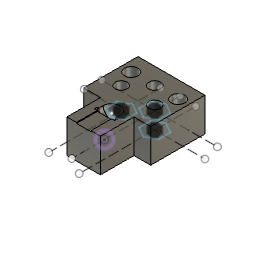
bending_tool_lower_LED v7 (Autodesk Fusion 360 design; units mm, degrees)
Autodesk Fusion 360 part; units mm, degrees
sketch "Skizze1" plane through (0, 0, 0) normal (0, 0, 1) x (1, 0, 0)
  line L0 (-3, 0) -> (-3, 0.8)
  line L1 (-3, 0.8) -> (-2.5, 0.8)
  line L2 (-2.5, 0.8) -> (-2.5, 2.1)
  line L3 (-8.4843, 2.1) -> (11.6981, 2.1) construction
  line L4 (0, 9) -> (0, -6.2163) construction
  arc A0 (0, 4.6) -> (-2.5, 2.1) centre (0, 2.1) ccw
  line L5 (0, 4.6) -> (0, 0)
  line L6 (0, 0) -> (-3, 0)
  line L7 (2.5, 2) -> (4.5, 2)
  line L8 (4.5, 2) -> (4.5, -2)
  line L9 (4.5, -2) -> (2.5, -2)
  line L10 (2.5, -2) -> (2.5, 2)
  line L11 (-4.5, 2) -> (-2.5, 2)
  line L12 (-2.5, 2) -> (-2.5, -2)
  line L13 (-2.5, -2) -> (-4.5, -2)
  line L14 (-4.5, -2) -> (-4.5, 2)
  point P0 (0, 2.1)
  dimension "d1" = 3
  dimension "d2" = 0.8
  dimension "d3" = 2.5
  dimension "d7" = 2.5
  dimension "d8" = 2
  dimension "d9" = 2
  dimension "d10" = 2
  dimension "d117" = 2.5
  dimension "d119" = 2
  dimension "d120" = 2
  dimension "d121" = 2
  dimension "d122" = 2.1
  dimension "d123" = 4.6
  constraint vertical L0
  constraint perpendicular L0 L1
  constraint perpendicular L1 L2
  constraint horizontal L3
  constraint perpendicular L3 L4
  constraint coincident L5.end L4
  constraint coincident L4 P0
  constraint coincident L3 P0
  constraint coincident L4 A0.start
  constraint coincident P0 A0.centre
  constraint coincident L5.end L6.start
  constraint perpendicular L0 L6
  constraint horizontal L7
  constraint vertical L8
  constraint horizontal L9
  constraint vertical L10
  constraint horizontal L11
  constraint vertical L12
  constraint horizontal L13
  constraint vertical L14
  constraint coincident L2.end L3
  measures "d1" distance of L5.end L0
  measures "d2" distance of L0.start L0.end
  measures "d3" distance of L5.end L2
  measures "d7" distance of L5.end L10
  measures "d8" vertical distance of L5.end L7.start
  measures "d9" distance of L5.end L9
  measures "d10" distance of L8 L10
  measures "d117" distance of L5.end L12
  measures "d119" distance of L12 L14
  measures "d120" distance of L5.end L13
  measures "d121" distance of L5.end L11
  measures "d122" distance of L5.end L3
  measures "d123" distance of L5.end A0.start
revolve "Drehen1" add sketch "Skizze1" angle 360 about axis through (0, 9, 0) along (0, -1, 0) contours L0 L1 L6 L12 | L2 A0 L5 L6 L12 makes body 1
sketch "Skizze2" plane through (0, 0, 0) normal (0, 0, 1) x (1, 0, 0)
  line L0 (-10, 20) -> (10, 20)
  line L1 (10, 20) -> (10, -6.2)
  line L2 (10, -6.2) -> (-10, -6.2)
  line L3 (-10, -6.2) -> (-10, 20)
  line L4 (0, 21.3723) -> (0, -17) construction
  line L5 (-26.2349, 0) -> (38.3962, 0) construction
  line L6 (5, -6.2) -> (5, 3.8)
  line L7 (5, 3.8) -> (10, 3.8)
  line L8 (-5, -6.2) -> (-5, 3.8)
  line L9 (-5, 3.8) -> (-10, 3.8)
  line L10 (-17, 10) -> (24.4562, 10) construction
  line L11 (-5, 26) -> (-5, 5) construction
  line L12 (5, 25.6741) -> (5, 5) construction
  circle A0 centre (-5, 10) radius 1.75
  circle A1 centre (5, 10) radius 1.75
  line L13 (-16, 15) -> (36.57, 15) construction
  circle A2 centre (0, 15) radius 1.75
  line L14 (-7, 22.2425) -> (-7, -4.6464) construction
  line L15 (7, 22.2425) -> (7, -3.3633) construction
  circle A3 centre (-7, 15) radius 2
  circle A4 centre (7, 15) radius 2
  dimension "d13" = 10
  dimension "d14" = 10
  dimension "d15" = 6.2
  dimension "d16" = 20
  dimension "d32" = 5
  dimension "d33" = 10
  dimension "d34" = 5
  dimension "d35" = 10
  dimension "d36" = 10
  dimension "d37" = 5
  dimension "d38" = 5
  dimension "d39" = 3.5
  dimension "d40" = 3.5
  dimension "d41" = 5
  dimension "d42" = 3.5
  dimension "d53" = 7
  dimension "d54" = 7
  constraint horizontal L0
  constraint vertical L1
  constraint horizontal L2
  constraint vertical L3
  constraint vertical L4
  constraint coincident L4 origin
  constraint horizontal L5
  constraint coincident origin L5
  constraint coincident L2 L6.start
  constraint perpendicular L2 L6
  constraint coincident L1 L7.end
  constraint perpendicular L1 L7
  constraint coincident L2 L8.start
  constraint perpendicular L5 L8
  constraint coincident L3 L9.end
  constraint perpendicular L3 L9
  constraint horizontal L10
  constraint vertical L11
  constraint perpendicular L0 L12
  constraint coincident L10 A0.centre
  constraint coincident L11 A0.centre
  constraint coincident L10 A1.centre
  constraint coincident L12 A1.centre
  constraint horizontal L13
  constraint coincident L13 A2.centre
  constraint coincident L4 A2.centre
  constraint perpendicular L9 L14
  constraint perpendicular L5 L15
  constraint coincident L13 A3.centre
  constraint coincident L14 A3.centre
  constraint tangent L11 A3
  constraint coincident L13 A4.centre
  constraint coincident L15 A4.centre
  constraint tangent L12 A4
  measures "d13" distance of L1 L4
  measures "d14" distance of L3 origin
  measures "d15" distance of L2 origin
  measures "d16" distance of L0 L5
  measures "d32" distance of L1 L6
  measures "d33" distance of L2 L7
  measures "d34" distance of L3 L8
  measures "d35" distance of L2 L9
  measures "d36" distance of L0 L10
  measures "d37" distance of L1 L12
  measures "d38" distance of L3 L11
  measures "d39" diameter of A1
  measures "d40" diameter of A0
  measures "d41" distance of L0 L13
  measures "d42" diameter of A2
  measures "d53" distance of origin L15
  measures "d54" distance of origin L14
extrude "Extrusion2" add sketch "Skizze2" against normal blind 10 separate body contours L0 L1 L2 L3 L6 L7 L8 L9 | A3 | A4 makes body 2
extrude "Extrusion7" cut sketch "Skizze2" against normal blind 5 contours A3 | A4 bodies 2
combine "Kombinieren1" operation cut target body 2 tool bodies 1
sketch "Skizze4" plane through (0, 0, 0) normal (0, 0, 1) x (1, 0, 0)
  line L0 (2.15, -6.2) -> (-2.15, -6.2)
  line L1 (-2.15, -6.2) -> (-2.15, 0)
  line L2 (-2.15, 0) -> (2.15, 0)
  line L3 (2.15, 0) -> (2.15, -6.2)
  line L4 (2.15, -6.2) -> (-2.15, 0) construction
  line L5 (-2.15, -6.2) -> (2.15, 0) construction
  line L6 (0, 9.7025) -> (0, -8.7035) construction
  line L7 (-7.2352, -6.2) -> (6.1757, -6.2) construction
  point P0 (0, -3.1)
  point P1 (0, -6.2)
  dimension "d21" = 4.3
  dimension "d22" = 6.2
  constraint horizontal L0
  constraint perpendicular L0 L1
  constraint parallel L0 L2
  constraint parallel L1 L3
  constraint coincident L4 P0
  constraint coincident L5 P0
  constraint vertical L6
  constraint coincident origin L6
  constraint coincident P0 L6
  constraint coincident origin L2
  constraint horizontal L7
  constraint coincident L6 P1
  constraint coincident L7 P1
  constraint coincident L0 P1
  measures "d21" distance of L0.start L0.end
  measures "d22" distance of origin L7
extrude "Extrusion4" cut sketch "Skizze4" against normal blind 0.25 bodies 2
ref_plane "Arbeitsebene1" through (0, 0, -6.5) normal (0, 0, 1) x (1, 0, 0)
sketch "Skizze7" plane through (0, 0, -6.5) normal (0, 0, 1) x (1, 0, 0)
  line L0 (-16.0259, 10) -> (20, 10) construction
  line L1 (-5, 21.68) -> (-5, -11.619) construction
  line L2 (5, 22.2413) -> (5, -12.5543) construction
  line L3 (-2.05, 11.7032) -> (-5, 13.4064)
  line L4 (-5, 13.4064) -> (-7.95, 11.7032)
  line L5 (-7.95, 11.7032) -> (-7.95, 8.2968)
  line L6 (-7.95, 8.2968) -> (-5, 6.5936)
  line L7 (-5, 6.5936) -> (-2.05, 8.2968)
  line L8 (-2.05, 8.2968) -> (-2.05, 11.7032)
  line L9 (7.95, 11.7032) -> (5, 13.4064)
  line L10 (5, 13.4064) -> (2.05, 11.7032)
  line L11 (2.05, 11.7032) -> (2.05, 8.2968)
  line L12 (2.05, 8.2968) -> (5, 6.5936)
  line L13 (5, 6.5936) -> (7.95, 8.2968)
  line L14 (7.95, 8.2968) -> (7.95, 11.7032)
  line L15 (-15.7752, 15) -> (18.7006, 15) construction
  line L16 (0, 22.633) -> (0, -9.7229) construction
  line L17 (2.95, 16.7032) -> (0, 18.4064)
  line L18 (0, 18.4064) -> (-2.95, 16.7032)
  line L19 (-2.95, 16.7032) -> (-2.95, 13.2968)
  line L20 (-2.95, 13.2968) -> (0, 11.5936)
  line L21 (0, 11.5936) -> (2.95, 13.2968)
  line L22 (2.95, 13.2968) -> (2.95, 16.7032)
  point P0 (-5, 10)
  point P1 (5, 10)
  point P2 (-5, 10)
  point P3 (5, 10)
  point P4 (0, 15)
  point P5 (0, 15)
  dimension "d44" = 10
  dimension "d45" = 5
  dimension "d46" = 5
  dimension "d47" = 5.9
  dimension "d48" = 5.9
  dimension "d51" = 15
  dimension "d52" = 5.9
  constraint horizontal L0
  constraint vertical L1
  constraint vertical L2
  constraint coincident L0 P2
  constraint coincident L1 P2
  constraint coincident L2 P3
  constraint coincident L0 P3
  constraint coincident P2 P0
  constraint coincident P3 P1
  constraint horizontal L15
  constraint vertical L16
  constraint coincident origin L16
  constraint coincident L15 P5
  constraint coincident L16 P5
  constraint coincident P5 P4
  measures "d44" distance of L0 origin
  measures "d45" distance of origin L2
  measures "d46" distance of origin L1
  measures "d47" distance of L11 L14
  measures "d48" distance of L5 L8
  measures "d51" distance of origin L15
  measures "d52" distance of L19 L22
extrude "Extrusion6" cut sketch "Skizze7" along normal blind 2.8 bodies 2
equation "d3 = d"
equation "d7 = d"
equation "d117 = d"
equation "d = 2.5 mm"
equation "d122 = 4.6 mm - d"
